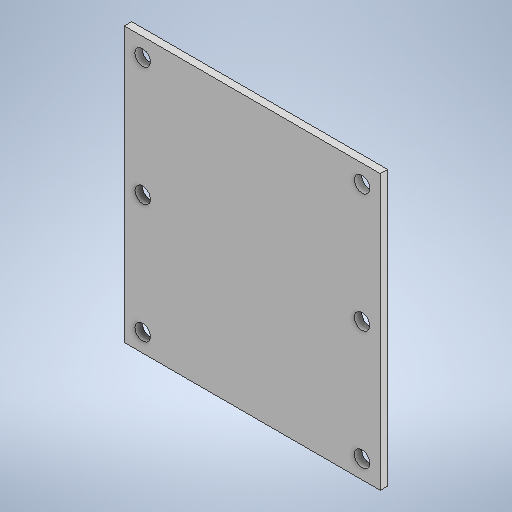
# Autodesk Inventor part: Ухо на швеллер пямое
Saved by Autodesk Inventor 2025 (Build 290162010, 162A)
## iProperties
Created: 2024-06-15
Part Number: Ухо на швеллер пямое
Material: Generic
Document SubType Name: Sheet Metal
Designer: admin
Density: 1 g/cm^3
Sheet Metal Rule: Default
Appearance: Default
Author: admin
Autodesk Inventor part; units mm, degrees
ref_plane "YZ Plane" through (0, 0, 0) normal (1, 0, 0) x (0, 1, 0)
ref_plane "XZ Plane" through (0, 0, 0) normal (0, 1, 0) x (-1, 0, 0)
ref_plane "XY Plane" through (0, 0, 0) normal (0, 0, 1) x (1, 0, 0)
sketch "Sketch1" plane through (0, 0, 0) normal (0, 1, 0) x (-1, 0, 0)
  line L0 (140, -150) -> (-140, -150)
  line L1 (-140, -150) -> (-140, 150)
  line L2 (-140, 150) -> (140, 150)
  line L3 (140, 150) -> (140, -150)
  line L4 (140, -150) -> (-140, 150) construction
  line L5 (-140, -150) -> (140, 150) construction
  point P0 (0, 0)
  point P1 (0, 0)
  dimension "d16" = 280
  dimension "d17" = 300
  measures "d16" distance of L1.end L2.end
  measures "d17" distance of L0.end L1.end
extrude "Plate1" add sketch "Sketch1" along normal blind 8
sketch "Sketch2" plane through (0, 0, 0) normal (0, -1, 0) x (1, 0, 0)
  line L0 (120, 130) -> (120, -130) construction
  line L1 (-140, -150) -> (140, -150) projected
  line L2 (140, -150) -> (140, 150) projected
  line L3 (140, 150) -> (-140, 150) projected
  line L4 (-140, 150) -> (-140, -150) projected
  point P0 (120, 0)
  point P1 (120, 0)
  point P2 (0, 0)
  dimension "d19" = 20
  dimension "d20" = 20
  constraints: 2 coincident, 2 end point, 1 horizontal alignment, 1 midpoint, 1 vertical
  measures "d19" distance between parallel lines of L2 L0
  measures "d20" distance from line of L0.start L3
hole "Hole1" at (120, 0, 130) at (120, 0, -130) at (120, 0, 0) direction (0, 1, 0) diameter 17 end through all
mirror "Mirror1" about plane through (0, 0, 0) normal (1, 0, 0) of "Hole1"
equation "\"d20\" = d19"
equation "\"d8\" = Thickness"
equation "\"d2\" = Thickness"
equation "\"BendRadius\" = Thickness"
equation "\"BendReliefWidth\" = Thickness"
equation "\"BendReliefDepth\" = 0.5 * Thickness"
equation "\"CornerReliefSize\" = 4 * Thickness"
equation "\"MinimumRemnant\" = 2 * Thickness"
equation "\"TransitionRadius\" = BendRadius"
equation "\"JacobiRadiusSize\" = BendRadius"
equation "\"GapSize\" = Thickness"
equation "\"Thickness\" = 8"
body "Solid1"
